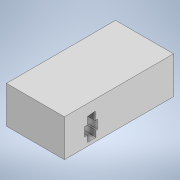
# Autodesk Inventor part: test blok
Saved by Autodesk Inventor 2020 (Build 240168000, 168)
## iProperties
Created: 2020-05-26
Part Number: test blok
Material: Generic
Document SubType Name: Modeling
Designer: Gebruiker
Density: 1 g/cm^3
Appearance: Default
Author: Gebruiker
Autodesk Inventor part; units mm, degrees
ref_plane "YZ Plane" through (0, 0, 0) normal (1, 0, 0) x (0, 1, 0)
ref_plane "XZ Plane" through (0, 0, 0) normal (0, 1, 0) x (-1, 0, 0)
ref_plane "XY Plane" through (0, 0, 0) normal (0, 0, 1) x (1, 0, 0)
sketch "Sketch1" plane through (0, 0, 0) normal (1, 0, 0) x (0, 1, 0)
  line L0 (10.9667, -32.2396) -> (-10.9667, -32.2396)
  line L1 (-10.9667, -32.2396) -> (-10.9667, 32.2396)
  line L2 (-10.9667, 32.2396) -> (10.9667, 32.2396)
  line L3 (10.9667, 32.2396) -> (10.9667, -32.2396)
  line L4 (10.9667, -32.2396) -> (-10.9667, 32.2396) construction
  line L5 (-10.9667, -32.2396) -> (10.9667, 32.2396) construction
  line L6 (-8.867, 14.9521) -> (-8.867, 18.6958)
  line L7 (-8.867, 18.6958) -> (-5.1781, 18.6958)
  line L8 (-5.1781, 18.6958) -> (-5.1781, 20.3884)
  line L9 (-5.1781, 20.3884) -> (0.0187, 20.3884)
  line L10 (0.0187, 20.3884) -> (0.0187, 18.6958)
  line L11 (0.0187, 18.6958) -> (4.2724, 18.6958)
  line L12 (4.2724, 18.6958) -> (4.8008, 14.1133)
  line L13 (4.8008, 14.1133) -> (0.0187, 14.1133)
  line L14 (0.0187, 14.1133) -> (0.0187, 12.7771)
  line L15 (0.0187, 12.7771) -> (-5.1781, 12.7771)
  line L16 (-5.1781, 12.7771) -> (-5.1781, 13.6309)
  line L17 (-5.1781, 13.6309) -> (-8.867, 13.6309)
  line L18 (-8.867, 13.6309) -> (-8.867, 14.9521)
  point P0 (0, 0)
  constraints: 38 end point, 8 point on line, 7 perpendicular, 3 parallel, 2 midpoint, 1 horizontal, 1 vertical
extrude "Extrusion1" add sketch "Sketch1" along normal blind 34.25
body "Solid1"
